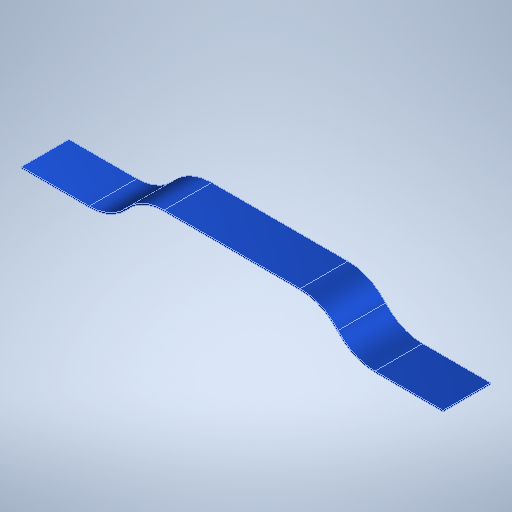
# Autodesk Inventor part: Кожух
Saved by Autodesk Inventor 2025 (Build 290162000, 162)
## iProperties
Created: 2025-02-24
Part Number: Кожух
Material: Алюминий 6061
Document SubType Name: Sheet Metal
Designer: volko
Density: 2.7 g/cm^3
Sheet Metal Rule: По умолчанию_мм
Appearance: Черный
Author: volko
Autodesk Inventor part; units mm, degrees
ref_plane "YZ Plane" through (0, 0, 0) normal (1, 0, 0) x (0, 1, 0)
ref_plane "XZ Plane" through (0, 0, 0) normal (0, 1, 0) x (-1, 0, 0)
ref_plane "XY Plane" through (0, 0, 0) normal (0, 0, 1) x (1, 0, 0)
sketch "Эскиз4" plane through (0, 0, 0) normal (0, 0, 1) x (1, 0, 0)
  line L0 (-310, 0) -> (-210, 0)
  arc A0 (-210, 0) -> (-155, 25) centre (-210, 73) ccw
  arc A1 (-100, 50) -> (-155, 25) centre (-100, -23) ccw
  line L1 (-100, 50) -> (0, 50)
  line L2 (0, -42.2) -> (0, 92.2)
  line L3 (310, 0) -> (210, 0)
  arc A2 (155, 25) -> (210, 0) centre (210, 73) ccw
  arc A3 (155, 25) -> (100, 50) centre (100, -23) ccw
  line L4 (100, 50) -> (0, 50)
  point P0 (0, 0)
  dimension "d39" = 50
  dimension "d61" = 100
  dimension "d63" = 200
  dimension "d64" = 620
  measures "d39" distance between parallel lines of L1 L0
  measures "d61" distance of L0.start L0.end
  measures "d63" distance of L4.start L1.start
  measures "d64" distance of L0.start L3.start
contour flange "Фланец по контуру2" sketch "Эскиз4" thickness 2 bend radius 2 width 70 along (0, 0, 1) mid plane no both sides yes wall seen from (260, 0, 0) lies toward (0, -1, 0) curves L3 A2 A3 L4 L1 A1 A0 L0
bend "Сгиб3"
corner "УглСтык3"
equation "\"d26\" = Толщина"
equation "\"d27\" = Ширина_просечки"
equation "\"d28\" = Глубина_просечки"
equation "\"d29\" = Мин_остаток"
equation "\"d30\" = Радиус_перехода"
equation "\"d32\" = Радиус_гибки"
equation "\"d34\" = Размер_просечки"
equation "\"d35\" = Размер_зазора"
equation "\"d36\" = Радиус_Якоби"
equation "\"Радиус_гибки\" = Толщина"
equation "\"Ширина_просечки\" = Толщина"
equation "\"Глубина_просечки\" = 0.5 * Толщина"
equation "\"Размер_просечки\" = 4 * Толщина"
equation "\"Мин_остаток\" = 2 * Толщина"
equation "\"Радиус_перехода\" = Радиус_гибки"
equation "\"Радиус_Якоби\" = Радиус_гибки"
equation "\"Размер_зазора\" = Толщина"
equation "\"Толщина\" = 2"
